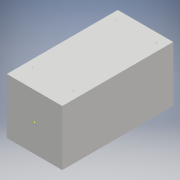
# Autodesk Inventor part: 垃圾桶外部
Saved by Autodesk Inventor 2017 (Build 210142000, 142)
## iProperties
Part Number: 垃圾桶外部
Material: 常规
Document SubType Name: Modeling
Designer: PANDA
Density: 1 g/cm^3
Appearance: 默认
Author: PANDA
Autodesk Inventor part; units mm, degrees
ref_plane "YZ Plane" through (0, 0, 0) normal (1, 0, 0) x (0, 1, 0)
ref_plane "XZ Plane" through (0, 0, 0) normal (0, 1, 0) x (-1, 0, 0)
ref_plane "XY Plane" through (0, 0, 0) normal (0, 0, 1) x (1, 0, 0)
sketch "草图1" plane through (0, 0, 0) normal (0, 1, 0) x (-1, 0, 0)
  line L0 (-150, -150) -> (150, -150)
  line L1 (150, -150) -> (150, 150)
  line L2 (150, 150) -> (-150, 150)
  line L3 (-150, 150) -> (-150, -150)
  point P0 (0, 0)
  dimension "d0" = 300
  dimension "d1" = 300
  constraints: 8 end point, 2 parallel, 1 horizontal, 1 perpendicular
  measures "d0" distance of L2.end L1.end
  measures "d1" distance of L1.end L0.end
extrude "拉伸1" add sketch "草图1" along normal blind 600
sketch "草图2" plane through (0, 600, 0) normal (0, 1, 0) x (1, 0, 0)
  line L0 (-140, -140) -> (140, -140)
  line L1 (140, -140) -> (140, 140)
  line L2 (140, 140) -> (-140, 140)
  line L3 (-140, 140) -> (-140, -140)
  point P0 (0, 0)
  dimension "d4" = 280
  dimension "d5" = 280
  constraints: 8 end point, 2 parallel, 1 horizontal, 1 perpendicular
  measures "d4" distance of L2.end L1.end
  measures "d5" distance of L1.end L0.end
extrude "拉伸2" cut sketch "草图2" along normal blind 550
sketch "草图3" plane through (0, 600, 0) normal (0, 1, 0) x (1, 0, 0)
  line L0 (-140, -140) -> (140, -140)
  line L1 (140, -140) -> (140, 140)
  line L2 (140, 140) -> (-140, 140)
  line L3 (-140, 140) -> (-140, -140)
  point P0 (0, 0)
  dimension "d8" = 280
  dimension "d9" = 280
  constraints: 8 end point, 2 parallel, 1 horizontal, 1 perpendicular
  measures "d8" distance of L2.end L1.end
  measures "d9" distance of L1.end L0.end
extrude "拉伸3" cut sketch "草图3" against normal blind 550
sketch "草图4" plane through (-150, 0, 150) normal (0, 0, 1) x (1, 0, 0)
  circle A0 centre (40, 100) radius 2
  point P0 (150, 0)
  dimension "d12" = 4
  constraints: 1 centre point
  measures "d12" diameter of A0
extrude "拉伸4" cut sketch "草图4" against normal through all
sketch "草图5" plane through (-150, 0, 150) normal (0, 0, 1) x (1, 0, 0)
  circle A0 centre (260, 100) radius 2
  circle A1 centre (40, 550) radius 2
  circle A2 centre (260, 550) radius 2
  point P0 (150, 0)
  constraints: 3 centre point
hole "孔1" at (110, 100, 150) direction (0, 0, -1) diameter 4 end through all
sketch "草图6" plane through (-150, 0, 150) normal (0, 0, 1) x (1, 0, 0)
  circle A0 centre (40, 550) radius 2
  point P0 (150, 0)
  constraints: 1 centre point
extrude "拉伸5" cut sketch "草图6" against normal through all
sketch "草图7" plane through (-150, 0, 150) normal (0, 0, 1) x (1, 0, 0)
  circle A0 centre (260, 550) radius 2
  point P0 (150, 0)
  dimension "d28" = 4
  constraints: 1 centre point
  measures "d28" diameter of A0
extrude "拉伸6" cut sketch "草图7" against normal through all
sketch "草图8" plane through (0, 0, 0) normal (0, -1, 0) x (1, 0, 0)
  point P0 (0, 0)
sketch "草图9" plane through (0, 50, 0) normal (0, 1, 0) x (1, 0, 0)
  line L0 (-140, -140) -> (140, -140)
  line L1 (140, -140) -> (140, 140)
  line L2 (140, 140) -> (-140, 140)
  line L3 (-140, 140) -> (-140, -140)
  point P0 (0, 0)
  dimension "d31" = 280
  dimension "d32" = 280
  constraints: 8 end point, 2 parallel, 1 horizontal, 1 perpendicular
  measures "d31" distance of L2.end L1.end
  measures "d32" distance of L1.end L0.end
extrude "拉伸7" cut sketch "草图9" against normal blind 30
sketch "草图10" plane through (0, 0, 0) normal (0, -1, 0) x (1, 0, 0)
  circle A0 centre (130, 130) radius 1.5
  circle A1 centre (-130, -130) radius 1.5
  circle A2 centre (130, -130) radius 1.5
  circle A3 centre (-130, 130) radius 1.5
  point P0 (0, 0)
  constraints: 4 centre point
sketch "草图11" plane through (0, 0, 0) normal (0, -1, 0) x (1, 0, 0)
  point P0 (0, 0)
hole "孔2" at (-130, 0, 130) direction (0, 1, 0) diameter 3 end through all
sketch "草图12" plane through (0, 0, 0) normal (0, -1, 0) x (1, 0, 0)
  point P0 (0, 0)
sketch "草图13" plane through (0, 0, 0) normal (0, -1, 0) x (1, 0, 0)
  circle A0 centre (130, 130) radius 1.5
  point P0 (0, 0)
  constraints: 1 centre point
hole "孔3" at (130, 0, 130) direction (0, 1, 0) diameter 3 end through all
sketch "草图14" plane through (0, 0, 0) normal (0, -1, 0) x (1, 0, 0)
  circle A0 centre (-130, -130) radius 1.5
  point P0 (0, 0)
  constraints: 1 centre point
hole "孔4" at (-130, 0, -130) direction (0, 1, 0) diameter 3 end through all
sketch "草图15" plane through (0, 0, 0) normal (0, -1, 0) x (1, 0, 0)
  circle A0 centre (130, -130) radius 1.5
  point P0 (0, 0)
  constraints: 1 centre point
hole "孔5" at (130, 0, -130) direction (0, 1, 0) diameter 3 end through all
